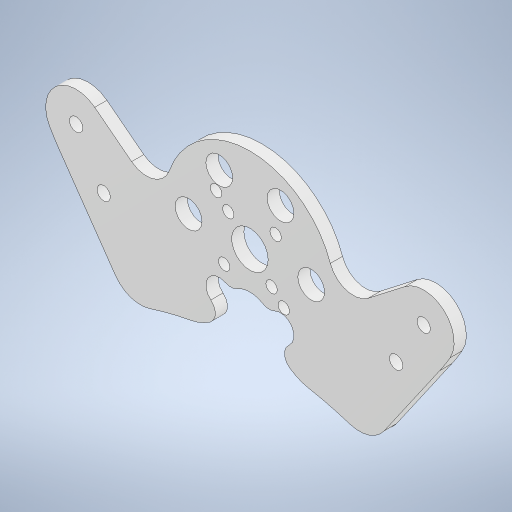
# Autodesk Inventor part: Support Ring
Saved by Autodesk Inventor 2023.2 (Build 272271000, 271)
## iProperties
Created: 2023-06-11
Part Number: Support Ring
Material: UHMW, White
Document SubType Name: Modeling
Designer: Nathan Cai
Mass: 8.45461 g
Surface Area: 73.3394 cm^2
Volume: 8.99426 cm^3
Density: 0.94 g/cm^3
Appearance: Smooth - White
Author: Nathan Cai
Autodesk Inventor part; units mm, degrees
ref_plane "YZ Plane" through (0, 0, 0) normal (1, 0, 0) x (0, 1, 0)
ref_plane "XZ Plane" through (0, 0, 0) normal (0, 1, 0) x (-1, 0, 0)
ref_plane "XY Plane" through (0, 0, 0) normal (0, 0, 1) x (1, 0, 0)
sketch "Sketch1" plane through (0, 0, 0) normal (0, 0, 1) x (1, 0, 0)
  circle A0 centre (0, 0) radius 60.325
  line L0 (0, 0) -> (0, 60.325) construction
  circle A1 centre (0, 52.3875) radius 7.9375 construction
  circle A2 centre (0, 52.3875) radius 1.7526
  circle A3 centre (-45.3689, -26.1937) radius 1.7526
  circle A4 centre (45.3689, -26.1938) radius 1.7526
  circle A5 centre (0, 0) radius 44.45
  circle A6 centre (0, -31.75) radius 28.575 construction
  circle A7 centre (0, -31.75) radius 28.575
  circle A8 centre (0, 0) radius 66.675
  line L1 (0, 0) -> (-33.3375, -57.7422)
  line L2 (0, 0) -> (33.3375, -57.7422)
  line L3 (-33.3375, -57.7422) -> (-49.5411, -34.4207)
  line L4 (33.3375, -57.7422) -> (49.5411, -34.4207)
  circle A9 centre (-45.3689, -26.1937) radius 7.9375 construction
  circle A10 centre (45.3689, -26.1938) radius 7.9375 construction
  circle A11 centre (0, 52.3875) radius 4.7625 construction
  circle A12 centre (-45.3689, -26.1937) radius 4.7625 construction
  circle A13 centre (45.3689, -26.1938) radius 4.7625 construction
  point P0 (-28.4756, -34.1313)
  point P1 (28.4756, -34.1313)
  point P2 (33.3375, -57.7422)
  point P3 (49.5411, -34.4207)
  dimension "d12" = 133.35
  dimension "d0" = 120.65
  dimension "d1" = 15.875
  dimension "d2" = 3.5052
  dimension "d5" = 360
  dimension "d7" = 88.9
  dimension "d10" = 57.15
  dimension "d11" = 57.15
  dimension "d13" = 30
  dimension "d17" = 360
  dimension "d21" = 9.525
  dimension "d24" = 360
  constraints: 13 centre point, 10 end point, 6 coincident, 3 tangent, 2 point on circle, 2 point on line, 2 symmetric about line, 1 vertical, 24 other
  measures "d0" diameter of A0
  measures "d1" diameter of A1
  measures "d2" diameter of A2
  measures "d7" diameter of A5
  measures "d10" diameter of A6
  measures "d11" diameter of A7
  measures "d13" angle of L0 L1
  measures "d21" diameter of A11
extrude "Extrusion1" add sketch "Sketch1" along normal blind 3.175 contours A0 L2 A7 A5 L1 | A0 L1 L3 | L4 L2 A0 | L1 A7 A0 | A0 L2 A8 L1 | A0 A7 L2 | A7 L1 A5 L2 | A7 A5 L1 | L2 A5 A7 | A7 L1 A5 | A5 A7 L2 L1 | L1 A7 L2 A5 | A5 L2 A7 | L1 L2 A7
fillet "Fillet1" radius 12.7 2 edges at (33.3375, -57.7422, 1.5875) (-33.3375, -57.7422, 1.5875)
sketch "Sketch2" plane through (0, 0, 0) normal (0, 0, -1) x (-1, 0, 0)
  point P0 (-38.1661, -38.1661)
  point P1 (-52.1358, -13.9698)
  point P2 (-13.9698, 52.1358)
  point P3 (13.9698, 52.1358)
  point P4 (52.1358, -13.9698)
  point P5 (38.1661, -38.1661)
hole "Hole1" at (38.1661, -38.1661, 0) at (52.1358, -13.9698, 0) at (13.9698, 52.1358, 0) at (-13.9698, 52.1358, 0) at (-52.1358, -13.9698, 0) at (-38.1661, -38.1661, 0) direction (0, 0, 1) diameter 3.5052 end through all
sketch "Sketch3" plane through (0, 0, 0) normal (0, 0, -1) x (-1, 0, 0)
  circle A0 centre (13.9698, 52.1358) radius 1.7526 projected
  circle A1 centre (13.9698, 52.1358) radius 7.9375
  circle A2 centre (-13.9698, 52.1358) radius 1.7526 projected
  circle A3 centre (-13.9698, 52.1358) radius 7.9375
  circle A4 centre (-52.1358, -13.9698) radius 7.9375
  circle A5 centre (-38.1661, -38.1661) radius 7.9375
  circle A6 centre (38.1661, -38.1661) radius 7.9375
  circle A7 centre (52.1358, -13.9698) radius 7.9375
  line L0 (20.8438, 56.1046) -> (59.0099, -10.001)
  line L1 (-59.0099, -10.001) -> (-20.8438, 56.1046)
  line L2 (38.1661, -46.1036) -> (-38.1661, -46.1036)
  arc A8 (44.3097, -15.2947) -> (8.9093, 46.0207) centre (-55.8649, -32.2536) ccw
  arc A9 (-8.9093, 46.0207) -> (-44.3097, -15.2947) centre (55.8649, -32.2536) ccw
  arc A10 (-35.4004, -30.726) -> (35.4004, -30.726) centre (0, 64.5072) ccw
  circle A11 centre (0, 0) radius 61.9125
  circle A12 centre (0, 52.3875) radius 1.7526 projected
  circle A13 centre (0, 52.3875) radius 7.9375
  line L3 (0, 52.3875) -> (0, 0) construction
  circle A14 centre (0, -31.75) radius 30.1625 construction
  circle A15 centre (-28.575, 15.9015) radius 1.7526
  circle A16 centre (-28.575, 15.9015) radius 26.9875 construction
  circle A17 centre (28.575, 15.9015) radius 1.7526
  circle A18 centre (0, -31.75) radius 4.7625
  circle A19 centre (0, -31.75) radius 9.5 construction
  circle A20 centre (0, -31.75) radius 8 construction
  line L4 (0, -31.75) -> (-6.7175, -25.0325) construction
  circle A21 centre (-6.7175, -25.0325) radius 1.5
  line L5 (0, -31.75) -> (6.7175, -25.0325) construction
  circle A22 centre (5.6569, -26.0931) radius 1.5
  circle A23 centre (0, -31.75) radius 12.5 construction
  circle A24 centre (8.8388, -22.9112) radius 1.5
  circle A25 centre (-8.8388, -40.5888) radius 1.5
  circle A26 centre (-5.6569, -37.4069) radius 1.5
  circle A27 centre (6.7175, -38.4675) radius 1.5
  circle A28 centre (0, -31.75) radius 16 construction
  circle A29 centre (0, -15.75) radius 3.5
  circle A30 centre (-8, -17.8936) radius 3.5
  circle A31 centre (-13.8564, -23.75) radius 3.5
  circle A32 centre (-16, -31.75) radius 3.5
  circle A33 centre (-13.8564, -39.75) radius 3.5
  circle A34 centre (-8, -45.6064) radius 3.5
  circle A35 centre (0, -31.75) radius 28.575
  circle A36 centre (0, -47.75) radius 3.5
  circle A37 centre (8, -45.6064) radius 3.5
  circle A38 centre (13.8564, -39.75) radius 3.5
  circle A39 centre (16, -31.75) radius 3.5
  circle A40 centre (13.8564, -23.75) radius 3.5
  circle A41 centre (8, -17.8936) radius 3.5
  point P0 (-44.3097, -15.2947)
  point P1 (-8.9093, 46.0207)
  point P2 (-16.0241, 59.8029)
  point P3 (-59.8029, -16.0241)
  point P4 (59.8029, -16.0241)
  point P5 (16.0241, 59.8029)
  dimension "d60" = 16
  dimension "d64" = 25
  dimension "d70" = 32
  dimension "d33" = 15.875
  dimension "d34" = 15.875
  dimension "d37" = 360
  dimension "d41" = 360
  dimension "d43" = 101.6
  dimension "d46" = 360
  dimension "d50" = 15.875
  dimension "d54" = 60.325
  dimension "d55" = 3.5052
  dimension "d56" = 28.575
  dimension "d57" = 53.975
  dimension "d58" = 9.525
  dimension "d59" = 19
  dimension "d61" = 45
  dimension "d62" = 3
  dimension "d63" = 3
  dimension "d65" = 3
  dimension "d68" = 360
  dimension "d71" = 7
  dimension "d74" = 360
  dimension "d85" = 57.15
  constraints: 36 centre point, 12 coincident, 12 end point, 12 point on circle, 7 tangent, 4 point on line, 1 perpendicular, 1 symmetric about line, 1 vertical, 1 vertical alignment, 83 other
  measures "d33" diameter of A1
  measures "d34" diameter of A3
  measures "d43" radius of A8
  measures "d50" diameter of A13
  measures "d54" diameter of A14
  measures "d55" diameter of A15
  measures "d56" distance from line of L3 A15.centre
  measures "d57" diameter of A16
  measures "d58" diameter of A18
  measures "d59" diameter of A19
  measures "d61" angle of L4 L3
  measures "d62" diameter of A21
  measures "d63" diameter of A22
  measures "d65" diameter of A24
  measures "d71" diameter of A29
  measures "d85" diameter of A35
extrude "Extrusion3" cut sketch "Sketch3" against normal through all contours A1 A11 A7 L0 | A3 L1 A4 A11
fillet "Fillet3" radius 12.7 4 edges at (-20.4179, 56.7645, 1.5875) (20.4179, 56.7645, 1.5875) (59.3685, -10.6998, 1.5875) (-59.3685, -10.6998, 1.5875)
extrude "Extrusion4" cut sketch "Sketch3" against normal through all contours A37 L2 | L2 A37 | A26 A10 | A10 A26 | A34 L2 | L2 A34 | A36 L2 | L2 A36 | A15 | A17 | A18 | A21 | A22 | A24 | A25 | A27 | A30 | A32 | A39 | A41
sketch "Sketch4" plane through (0, 0, 3.175) normal (0, 0, 1) x (1, 0, 0)
  circle A0 centre (0, -31.75) radius 4.7625 projected
  circle A1 centre (8.8388, -40.5888) radius 1.5 projected
  circle A2 centre (6.7175, -25.0325) radius 1.5 projected
  circle A3 centre (-5.6569, -26.0931) radius 1.5 projected
  circle A4 centre (-28.575, 15.9015) radius 1.7526 projected
  circle A5 centre (8, -45.6064) radius 3.5 projected
  circle A6 centre (5.6569, -37.4069) radius 1.5 projected
  circle A7 centre (-6.7175, -38.4675) radius 1.5 projected
  circle A8 centre (16, -31.75) radius 3.5 projected
  circle A9 centre (8, -17.8936) radius 3.5 projected
  circle A10 centre (-8.8388, -22.9112) radius 1.5 projected
  circle A11 centre (28.575, 15.9015) radius 1.7526 projected
  arc A12 (-56.9, -6.3464) -> (-58.1418, -16.0821) centre (-45.9014, -12.6964) ccw projected
  arc A13 (-58.1418, -16.0821) -> (-49.5411, -34.4207) centre (0, 0) ccw projected
  line L0 (-49.5411, -34.4207) -> (-35.0482, -55.2801) projected
  arc A14 (-35.0482, -55.2801) -> (-30.411, -59.3357) centre (-24.6185, -48.0337) ccw projected
  arc A15 (-30.411, -59.3357) -> (30.411, -59.3357) centre (0, 0) ccw projected
  arc A16 (30.411, -59.3357) -> (35.0482, -55.2801) centre (24.6185, -48.0337) ccw projected
  line L1 (35.0482, -55.2801) -> (49.5411, -34.4207) projected
  arc A17 (49.5411, -34.4207) -> (58.1418, -16.0821) centre (0, 0) ccw projected
  arc A18 (58.1418, -16.0821) -> (56.9, -6.3464) centre (45.9014, -12.6964) ccw projected
  line L2 (56.9, -6.3464) -> (22.9538, 52.45) projected
  arc A19 (22.9538, 52.45) -> (15.1434, 58.3934) centre (11.9553, 46.1) ccw projected
  arc A20 (15.1434, 58.3934) -> (-15.1434, 58.3934) centre (0, 0) ccw projected
  arc A21 (-15.1434, 58.3934) -> (-22.9538, 52.45) centre (-11.9553, 46.1) ccw projected
  line L3 (-22.9538, 52.45) -> (-56.9, -6.3464) projected
  circle A22 centre (-52.1358, -13.9698) radius 1.7526 projected
  circle A23 centre (13.9698, 52.1358) radius 1.7526 projected
  circle A24 centre (38.1661, -38.1661) radius 1.7526 projected
  circle A25 centre (52.1358, -13.9698) radius 1.7526 projected
  circle A26 centre (-13.9698, 52.1358) radius 1.7526 projected
  circle A27 centre (-38.1661, -38.1661) radius 1.7526 projected
  circle A28 centre (0, 52.3875) radius 1.7526 projected
  circle A29 centre (-45.3689, -26.1937) radius 1.7526 projected
  circle A30 centre (45.3689, -26.1938) radius 1.7526 projected
  arc A31 (-39.0154, -13.4694) -> (-33.8965, -23.551) centre (0, 0) ccw
  line L4 (-33.8965, -23.551) -> (-20.3396, -43.0632)
  arc A32 (-20.3396, -43.0632) -> (20.3396, -43.0632) centre (0, 0) ccw
  line L5 (20.3396, -43.0632) -> (33.8965, -23.551)
  arc A33 (33.8965, -23.551) -> (39.0154, -13.4694) centre (0, 0) ccw
  line L6 (39.0154, -13.4694) -> (7.8428, 40.523)
  arc A34 (7.8428, 40.523) -> (-7.8428, 40.523) centre (0, 0) ccw
  line L7 (-7.8428, 40.523) -> (-39.0154, -13.4694)
  circle A35 centre (0, -31.75) radius 22.225
  circle A36 centre (-28.575, 15.9015) radius 1.7526 projected
  circle A37 centre (-28.575, 15.9015) radius 9.525
  circle A38 centre (28.575, 15.9015) radius 1.7526 projected
  circle A39 centre (28.575, 15.9015) radius 9.525
  point P0 (-24.9713, -36.3969)
  point P1 (24.9713, -36.3969)
  point P2 (27.5238, 6.4346)
  point P3 (19.8509, 19.7244)
  point P4 (-19.8509, 19.7244)
  point P5 (-27.5238, 6.4346)
  point P6 (-18.6651, -43.815)
  point P7 (18.6651, -43.815)
  dimension "d78" = 19.05
  dimension "d79" = 44.45
  dimension "d80" = 19.05
  dimension "d81" = 19.05
  constraints: 8 end point, 8 point on circle, 7 centre point, 3 coincident, 7 other
  measures "d78" distance between parallel lines of L3 L7
  measures "d79" diameter of A35
  measures "d80" diameter of A37
  measures "d81" diameter of A39
extrude "Extrusion5" cut sketch "Sketch4" against normal through all contours A32 L4 A31 L7 A37 A34 L6 A39 A33 L5 A35 | L7 A37 | A39 L6 picked at (-22.3629, 12.124) picked at (23.5795, 11.3625)
fillet "Fillet4" radius 6.35 8 edges at (-7.8428, 40.523, 1.5875) (7.8428, 40.523, 1.5875) (-39.0154, -13.4694, 1.5875) (39.0154, -13.4694, 1.5875) (18.6651, -43.815, 1.5875) (-18.6651, -43.815, 1.5875) (-20.3396, -43.0632, 1.5875) (20.3396, -43.0632, 1.5875)
sketch "Sketch5" plane through (0, 0, 3.175) normal (0, 0, 1) x (1, 0, 0)
  circle A0 centre (-28.575, 15.9015) radius 1.7526 projected
  circle A1 centre (-28.575, 15.9015) radius 7.9375
  circle A2 centre (28.575, 15.9015) radius 1.7526 projected
  circle A3 centre (28.575, 15.9015) radius 7.9375
  circle A4 centre (13.9698, 52.1358) radius 1.7526 projected
  circle A5 centre (13.9698, 52.1358) radius 7.9375
  circle A6 centre (-13.9698, 52.1358) radius 1.7526 projected
  circle A7 centre (-13.9698, 52.1358) radius 7.9375
  circle A8 centre (-52.1358, -13.9698) radius 1.7526 projected
  circle A9 centre (-52.1358, -13.9698) radius 7.9375
  circle A10 centre (52.1358, -13.9698) radius 1.7526 projected
  circle A11 centre (52.1358, -13.9698) radius 7.9375
  arc A12 (-57.6186, -8.2301) -> (-21.6818, 54.0142) centre (-146.0018, 84.2942) ccw
  circle A13 centre (0, 52.3875) radius 1.7526 projected
  line L0 (0, 0) -> (0, 52.3875) construction
  arc A14 (21.6818, 54.0142) -> (57.6186, -8.2301) centre (146.0018, 84.2942) ccw
  arc A15 (0, -54.1) -> (-26.1235, -58.2352) centre (0, -138.6838) ccw
  circle A16 centre (16, -31.75) radius 3.5 projected
  circle A17 centre (0, -47.75) radius 6.35
  circle A18 centre (-28.575, -50.6857) radius 7.9375
  line L1 (-49.5411, -34.4207) -> (-35.0482, -55.2801) projected
  arc A19 (26.1235, -58.2352) -> (0, -54.1) centre (0, -138.6838) ccw
  circle A20 centre (28.575, -50.6857) radius 7.9375
  line L2 (-32.2042, -25.9868) -> (-33.8965, -23.551) projected
  arc A21 (-37.8102, -16.5534) -> (-33.8965, -23.551) centre (0, 0) ccw projected
  arc A22 (-37.4925, -10.8317) -> (-37.8102, -16.5534) centre (-31.9932, -14.0067) ccw projected
  line L3 (-37.4925, -10.8317) -> (-9.3657, 37.8853) projected
  arc A23 (-4.5694, 41.0213) -> (-9.3657, 37.8853) centre (-3.8664, 34.7103) ccw projected
  arc A24 (4.5694, 41.0213) -> (-4.5694, 41.0213) centre (0, 0) ccw projected
  arc A25 (9.3657, 37.8853) -> (4.5694, 41.0213) centre (3.8664, 34.7103) ccw projected
  line L4 (9.3657, 37.8853) -> (37.4925, -10.8317) projected
  arc A26 (37.8102, -16.5534) -> (37.4925, -10.8317) centre (31.9932, -14.0067) ccw projected
  arc A27 (33.8965, -23.551) -> (37.8102, -16.5534) centre (0, 0) ccw projected
  line L5 (33.8965, -23.551) -> (32.2042, -25.9868) projected
  arc A28 (20.9917, -24.4494) -> (32.2042, -25.9868) centre (26.9893, -22.3635) ccw projected
  arc A29 (20.9917, -24.4494) -> (-20.9917, -24.4494) centre (0, -31.75) ccw projected
  arc A30 (-32.2042, -25.9868) -> (-20.9917, -24.4494) centre (-26.9893, -22.3635) ccw projected
  circle A31 centre (0, -31.75) radius 4.7625 projected
  circle A32 centre (8.8388, -40.5888) radius 1.5 projected
  circle A33 centre (6.7175, -25.0325) radius 1.5 projected
  circle A34 centre (-5.6569, -26.0931) radius 1.5 projected
  circle A35 centre (-28.575, 15.9015) radius 1.7526 projected
  circle A36 centre (8, -45.6064) radius 3.5 projected
  circle A37 centre (5.6569, -37.4069) radius 1.5 projected
  circle A38 centre (-6.7175, -38.4675) radius 1.5 projected
  circle A39 centre (16, -31.75) radius 3.5 projected
  circle A40 centre (8, -17.8936) radius 3.5 projected
  circle A41 centre (-8.8388, -22.9112) radius 1.5 projected
  circle A42 centre (28.575, 15.9015) radius 1.7526 projected
  arc A43 (-56.9, -6.3464) -> (-58.1418, -16.0821) centre (-45.9014, -12.6964) ccw projected
  arc A44 (-58.1418, -16.0821) -> (-49.5411, -34.4207) centre (0, 0) ccw projected
  line L6 (-49.5411, -34.4207) -> (-35.0482, -55.2801) projected
  arc A45 (-35.0482, -55.2801) -> (-30.411, -59.3357) centre (-24.6185, -48.0337) ccw projected
  arc A46 (-30.411, -59.3357) -> (30.411, -59.3357) centre (0, 0) ccw projected
  arc A47 (30.411, -59.3357) -> (35.0482, -55.2801) centre (24.6185, -48.0337) ccw projected
  line L7 (35.0482, -55.2801) -> (49.5411, -34.4207) projected
  arc A48 (49.5411, -34.4207) -> (58.1418, -16.0821) centre (0, 0) ccw projected
  arc A49 (58.1418, -16.0821) -> (56.9, -6.3464) centre (45.9014, -12.6964) ccw projected
  line L8 (56.9, -6.3464) -> (22.9538, 52.45) projected
  arc A50 (22.9538, 52.45) -> (15.1434, 58.3934) centre (11.9553, 46.1) ccw projected
  arc A51 (15.1434, 58.3934) -> (-15.1434, 58.3934) centre (0, 0) ccw projected
  arc A52 (-15.1434, 58.3934) -> (-22.9538, 52.45) centre (-11.9553, 46.1) ccw projected
  line L9 (-22.9538, 52.45) -> (-56.9, -6.3464) projected
  circle A53 centre (-52.1358, -13.9698) radius 1.7526 projected
  circle A54 centre (13.9698, 52.1358) radius 1.7526 projected
  circle A55 centre (38.1661, -38.1661) radius 1.7526 projected
  circle A56 centre (52.1358, -13.9698) radius 1.7526 projected
  circle A57 centre (-13.9698, 52.1358) radius 1.7526 projected
  circle A58 centre (-38.1661, -38.1661) radius 1.7526 projected
  circle A59 centre (0, 52.3875) radius 1.7526 projected
  circle A60 centre (-45.3689, -26.1937) radius 1.7526 projected
  circle A61 centre (45.3689, -26.1938) radius 1.7526 projected
  line L10 (6.35, -47.75) -> (6.35, -54.3387)
  line L11 (-6.35, -47.75) -> (-6.35, -54.3387)
  circle A62 centre (-45.3689, -26.1937) radius 1.7526 projected
  circle A63 centre (-45.3689, -26.1937) radius 7.9375
  circle A64 centre (45.3689, -26.1938) radius 1.7526 projected
  circle A65 centre (45.3689, -26.1938) radius 7.9375
  line L12 (-25.9508, -31.2029) -> (-45.0002, -16.4366)
  line L13 (20.9707, -35.0634) -> (41.2015, -19.3812)
  arc A66 (20.9917, -24.4494) -> (32.2042, -25.9868) centre (26.9893, -22.3635) ccw projected
  point P0 (35.0936, -55.2148)
  point P1 (-35.0936, -55.2148)
  point P2 (21.5826, 54.3829)
  point P3 (57.6186, -8.2301)
  point P4 (57.8882, -8.5004)
  point P5 (-57.8882, -8.5004)
  point P6 (-21.5826, 54.3829)
  point P7 (-52.243, -30.1625)
  point P8 (-40.506, -19.9203)
  point P9 (-30.8797, -27.3823)
  point P10 (30.8797, -27.3823)
  point P11 (40.506, -19.9203)
  point P12 (52.243, -30.1625)
  dimension "d89" = 15.875
  dimension "d90" = 15.875
  dimension "d93" = 15.875
  dimension "d86" = 15.875
  dimension "d87" = 15.875
  dimension "d88" = 15.875
  dimension "d91" = 15.875
  dimension "d92" = 12.7
  dimension "d94" = 28.575
  dimension "d99" = 15.875
  dimension "d100" = 15.875
  constraints: 11 centre point, 11 point on circle, 10 end point, 8 coincident, 7 symmetric about line, 7 tangent, 3 vertical, 1 point on line, 19 other
  measures "d86" diameter of A1
  measures "d87" diameter of A3
  measures "d88" diameter of A5
  measures "d91" diameter of A11
  measures "d92" diameter of A17
  measures "d94" horizontal distance of L0.start point (-28.575, -50.686)
  measures "d99" diameter of A63
  measures "d100" diameter of A65
extrude "Extrusion6" cut sketch "Sketch5" against normal through all contours L3 A1 | A1 A12 A7 A51 A5 A14 A3 L4 A25 A24 A23 L3 | L3 A22 A21 L2 A30 L12 A9 A12 A1 | A12 A9 A43 L9 A52 A7 | A9 A63 A44 A43 | A7 A52 A51 | L12 A63 A9 | A9 A63 A44 | A51 A50 A5 | A3 L4 | A50 L8 A49 A11 A14 A5 | A14 A11 A65 L13 A28 L5 A27 A26 L4 A3 | A11 A49 A48 A65 | A11 A48 A65 | A19 A20 A47 A46 A45 A18 A15 | A15 L11 A17 | A17 A36 | A17 A36 L10 A19 | A36 A17 | A17 L10 A36 picked at (-24.7993, 13.7487) picked at (-11.4351, 57.0317) picked at (11.4163, 57.0172) picked at (24.7993, 13.7487) picked at (6.3379, -48.3675)
fillet "Fillet5" radius 12.7 2 edges at (-6.35, -54.3387, 1.5875) (6.35, -54.3387, 1.5875)
fillet "Fillet6" radius 3.175 4 edges at (-4.9892, -43.8218, 1.5875) (4.9892, -43.8218, 1.5875) (6.35, -48.6931, 1.5875) (-6.35, -48.6931, 1.5875)
body "Solid1"
